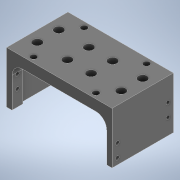
# Autodesk Inventor part: Carriage
Saved by Autodesk Inventor 2022 (Build 260153000, 153)
## iProperties
Created: 2021-06-15
Part Number: Carriage
Material: Generic
Document SubType Name: Modeling
Designer: burgessb
Density: 1 g/cm^3
Appearance: Gray
Author: burgessb
Autodesk Inventor part; units mm, degrees
ref_plane "YZ Plane" through (0, 0, 0) normal (1, 0, 0) x (0, 1, 0)
ref_plane "XZ Plane" through (0, 0, 0) normal (0, 1, 0) x (-1, 0, 0)
ref_plane "XY Plane" through (0, 0, 0) normal (0, 0, 1) x (1, 0, 0)
sketch "Sketch1" plane through (0, 0, 0) normal (0, 1, 0) x (-1, 0, 0)
  line L0 (-45, 17.5) -> (45, 17.5)
  line L1 (45, 17.5) -> (45, -17.5)
  line L2 (45, -17.5) -> (-45, -17.5)
  line L3 (-45, -17.5) -> (-45, 17.5)
  line L4 (-45, 17.5) -> (45, -17.5) construction
  line L5 (45, 17.5) -> (-45, -17.5) construction
  circle A0 centre (-39, 10) radius 2.25
  circle A1 centre (-11, 10) radius 2.25
  circle A2 centre (-11, -10) radius 2.25
  circle A3 centre (-39, -10) radius 2.25
  line L6 (0, 17.5) -> (0, -17.5) construction
  circle A4 centre (39, 10) radius 2.25
  circle A5 centre (11, 10) radius 2.25
  circle A6 centre (11, -10) radius 2.25
  circle A7 centre (39, -10) radius 2.25
  point P0 (0, 0)
  dimension "d0" = 90
  dimension "d1" = 35
  dimension "d12" = 4.5
  dimension "d13" = 4.5
  dimension "d14" = 4.5
  dimension "d15" = 4.5
  dimension "d16" = 0
  dimension "d17" = 0
  dimension "d18" = 0
  dimension "d19" = 0
  dimension "d21" = 10
  dimension "d22" = 20
  dimension "d23" = 28
  dimension "d50" = 50
  constraints: 14 end point, 8 centre point, 4 midpoint, 4 symmetric about line, 2 parallel, 1 horizontal, 1 perpendicular, 4 other
  measures "d0" distance of L1.end L2.end
  measures "d1" distance of L0.end L1.end
  measures "d12" diameter of A0
  measures "d13" diameter of A1
  measures "d14" diameter of A2
  measures "d15" diameter of A3
  measures "d16" horizontal distance of A2.centre A1.centre
  measures "d17" vertical distance of A3.centre A2.centre
  measures "d18" horizontal distance of A3.centre A0.centre
  measures "d19" vertical distance of A0.centre A1.centre
  measures "d21" vertical distance of point (0, 0) A1.centre
  measures "d22" distance of A2.centre A1.centre
  measures "d23" distance of A2.centre A3.centre
  measures "d50" distance of A6.centre A3.centre
extrude "Extrusion1" add sketch "Sketch1" along normal blind 8
sketch "Sketch2" plane through (0, 8, 0) normal (0, 1, 0) x (1, 0, 0)
  line L0 (45, 17.5) -> (-45, 17.5) projected
  line L1 (-45, 17.5) -> (-45, -17.5) projected
  line L2 (-45, -17.5) -> (45, -17.5) projected
  line L3 (45, -17.5) -> (45, 17.5) projected
  line L4 (46, -18.5) -> (-46, -18.5)
  line L5 (-46, -18.5) -> (-46, 18.5)
  line L6 (-46, 18.5) -> (46, 18.5)
  line L7 (46, 18.5) -> (46, -18.5)
  line L8 (49, -28.5) -> (49, 28.5)
  line L9 (49, -28.5) -> (44, -28.5)
  line L10 (44, -28.5) -> (44, -18.5)
  line L11 (49, 28.5) -> (44, 28.5)
  line L12 (44, 28.5) -> (44, 18.5)
  line L13 (44, -18.5) -> (44, -17.5)
  line L14 (-45, -17.5) -> (45, -17.5) projected
  line L15 (44, 18.5) -> (44, 17.5)
  line L16 (45, 17.5) -> (-45, 17.5) projected
  line L17 (0, -21.8029) -> (0, 22.7316) construction
  line L18 (-49, -28.5) -> (-49, 28.5)
  line L19 (-49, -28.5) -> (-44, -28.5)
  line L20 (-44, -28.5) -> (-44, -18.5)
  line L21 (-49, 28.5) -> (-44, 28.5)
  line L22 (-44, 28.5) -> (-44, 18.5)
  line L23 (-44, -18.5) -> (-44, -17.5)
  line L24 (-44, 18.5) -> (-44, 17.5)
  point P0 (0, 0)
  point P1 (-44, 17.5)
  dimension "d4" = 1
  dimension "d5" = 3
  dimension "d6" = 10
  dimension "d7" = 10
  dimension "d8" = 5
  dimension "d9" = 5
  dimension "d24" = 0
  constraints: 38 end point, 10 point on line, 8 symmetric about line, 2 perpendicular, 2 vertical, 1 horizontal, 3 other
  measures "d4" distance between parallel lines of L2 L4
  measures "d5" distance between parallel lines of L8 L7
  measures "d6" vertical distance of L6.end L8.end
  measures "d7" vertical distance of L4.start L8.start
  measures "d8" distance of L8.start L9.end
  measures "d9" distance of L8.end L11.end
  measures "d24" distance from line of point (0, 0) L17
extrude "Extrusion2" add sketch "Sketch2" against normal blind 8 contours L0 L15 L6 L7 L4 L13 L2 L3 | L0 L1 L2 L23 L4 L5 L6 L24 | L12 L11 L8 L9 L10 L4 L7 L6 | L6 L5 L4 L20 L19 L18 L21 L22
sketch "Sketch3" plane through (0, 0, 0) normal (0, -1, 0) x (1, 0, 0)
  line L0 (44, -17.5) -> (44, -28.5) projected
  line L1 (44, -28.5) -> (49, -28.5) projected
  line L2 (49, -28.5) -> (49, 28.5) projected
  line L3 (49, 28.5) -> (44, 28.5) projected
  line L4 (44, 28.5) -> (44, 17.5) projected
  line L5 (-44, 17.5) -> (44, 17.5) projected
  line L6 (-44, 17.5) -> (-44, 28.5) projected
  line L7 (-44, 28.5) -> (-49, 28.5) projected
  line L8 (-49, 28.5) -> (-49, -28.5) projected
  line L9 (-49, -28.5) -> (-44, -28.5) projected
  line L10 (-44, -28.5) -> (-44, -17.5) projected
  line L11 (44, -17.5) -> (-44, -17.5) projected
  circle A0 centre (-11, -10) radius 2.25 projected
  circle A1 centre (-11, 10) radius 2.25 projected
  circle A2 centre (-39, 10) radius 2.25 projected
  circle A3 centre (-39, -10) radius 2.25 projected
  circle A4 centre (39, -10) radius 2.25 projected
  circle A5 centre (11, -10) radius 2.25 projected
  circle A6 centre (11, 10) radius 2.25 projected
  circle A7 centre (39, 10) radius 2.25 projected
  line L12 (-45, -17.5) -> (45, -17.5)
  line L13 (45, -17.5) -> (45, 17.5)
  line L14 (45, 17.5) -> (-45, 17.5)
  line L15 (-45, 17.5) -> (-45, -17.5)
  line L16 (-45, -17.5) -> (45, 17.5) construction
  line L17 (45, -17.5) -> (-45, 17.5) construction
  line L18 (-46, -18.5) -> (46, -18.5)
  line L19 (46, -18.5) -> (46, 18.5)
  line L20 (46, 18.5) -> (-46, 18.5)
  line L21 (-46, 18.5) -> (-46, -18.5)
  line L22 (-44, 17.5) -> (-44, 18.5)
  line L23 (-44, -17.5) -> (-44, -18.5)
  line L24 (44, -17.5) -> (-44, -17.5) projected
  line L25 (44, -17.5) -> (44, -18.5)
  line L26 (44, 17.5) -> (44, 18.5)
  point P0 (0, 0)
  point P1 (44, 18.5)
  point P2 (44, -18.5)
  point P3 (-44, -18.5)
  point P4 (-44, 18.5)
  dimension "d26" = 35
  dimension "d27" = 1
  dimension "d52" = 90
  constraints: 28 end point, 4 parallel, 4 perpendicular, 4 point on line, 2 midpoint, 2 vertical, 1 horizontal, 3 other
  measures "d26" distance of L13.end L12.end
  measures "d27" distance between parallel lines of L15 L21
  measures "d52" distance of L13.end L14.end
extrude "Extrusion3" add sketch "Sketch3" along normal blind 30 contours L18 L19 L20 L4 L3 L2 L1 L0 | L10 L9 L8 L7 L6 L20 L21 L18
sketch "Sketch4" plane through (49, 8, 28.5) normal (1, 0, 0) x (0, 0, -1)
  circle A0 centre (5, -32.5) radius 1.65
  circle A1 centre (5, -20.5) radius 1.65
  line L0 (0, 0) -> (57, 0) projected
  line L1 (0, 0) -> (0, -38) projected
  line L2 (57, 0) -> (57, -38) projected
  circle A2 centre (52, -23.5) radius 1.65
  circle A3 centre (52, -11.5) radius 1.65
  line L3 (57, -38) -> (0, -38) projected
  line L4 (16.25, -8) -> (20.75, -8) projected
  line L5 (16.25, -8) -> (20.75, -8) projected
  line L6 (36.25, -8) -> (40.75, -8) projected
  line L7 (36.25, -8) -> (40.75, -8) projected
  line L8 (36.25, -8) -> (40.75, -8) projected
  line L9 (16.25, -8) -> (20.75, -8) projected
  line L10 (16.25, -8) -> (20.75, -8) projected
  line L11 (36.25, -8) -> (40.75, -8) projected
  line L12 (47, -8) -> (10, -8) projected
  line L13 (10, -8) -> (11, -8) projected
  line L14 (11, -8) -> (10, -8) projected
  line L15 (10, -8) -> (47, -8) projected
  line L16 (47, -8) -> (46, -8) projected
  line L17 (46, -8) -> (47, -8) projected
  line L18 (19.0432, -26.5) -> (-6.642, -26.5)
  point P0 (28.5, -8)
  dimension "d30" = 3.3
  dimension "d31" = 3.3
  dimension "d33" = 12
  dimension "d34" = 0
  dimension "d36" = 5
  dimension "d39" = 3.3
  dimension "d40" = 3.3
  dimension "d41" = 12
  dimension "d42" = 0
  dimension "d43" = 5
  dimension "d53" = 9
  dimension "d54" = 18.5
  dimension "d55" = 6
  dimension "d56" = 6
  constraints: 4 centre point, 2 end point, 1 horizontal
  measures "d30" diameter of A0
  measures "d31" diameter of A1
  measures "d33" distance of A0.centre A1.centre
  measures "d34" horizontal distance of A0.centre A1.centre
  measures "d36" distance from line of L1 A0.centre
  measures "d39" diameter of A2
  measures "d40" diameter of A3
  measures "d41" distance of A2.centre A3.centre
  measures "d42" horizontal distance of A2.centre A3.centre
  measures "d43" distance from line of L2 A2.centre
  measures "d53" vertical distance of A3.centre A1.centre
  measures "d54" distance between parallel lines of L18 L12
  measures "d55" distance from line of L18 A1.centre
  measures "d56" distance from line of L18 A0.centre
extrude "Extrusion4" cut sketch "Sketch4" against normal up to surface (5 mm away) contours A0 | A1 | A2 | A3
sketch "Sketch5" plane through (-49, 8, -28.5) normal (-1, 0, 0) x (0, 0, 1)
  line L0 (0, 0) -> (11, 0) projected
  line L1 (0, 0) -> (0, -38) projected
  line L2 (11, 0) -> (11, -8) projected
  line L3 (46, 0) -> (57, 0) projected
  line L4 (46, -8) -> (46, 0) projected
  line L5 (57, 0) -> (57, -38) projected
  line L6 (57, 0) -> (0, 0) projected
  line L7 (28.5, 0) -> (28.5, -38) construction
  line L8 (57, -38) -> (0, -38) projected
  line L9 (47, -8) -> (46, -8) projected
  line L10 (11, -8) -> (10, -8) projected
  line L11 (57, -38) -> (47, -38) projected
  line L12 (10, -38) -> (0, -38) projected
  line L13 (47, -8) -> (47, -38) projected
  line L14 (10, -8) -> (10, -38) projected
  circle A0 centre (5, -23.5) radius 1.65 projected
  circle A1 centre (5, -23.5) radius 1.65 projected
  circle A2 centre (5, -11.5) radius 1.65 projected
  circle A3 centre (5, -11.5) radius 1.65 projected
  circle A4 centre (52, -32.5) radius 1.65 projected
  circle A5 centre (52, -32.5) radius 1.65 projected
  circle A6 centre (52, -20.5) radius 1.65 projected
  circle A7 centre (52, -20.5) radius 1.65 projected
  circle A8 centre (52, -23.5) radius 1.65
  circle A9 centre (52, -23.5) radius 1.65
  circle A10 centre (52, -11.5) radius 1.65
  circle A11 centre (52, -11.5) radius 1.65
  circle A12 centre (5, -32.5) radius 1.65
  circle A13 centre (5, -32.5) radius 1.65
  circle A14 centre (5, -20.5) radius 1.65
  circle A15 centre (5, -20.5) radius 1.65
  point P0 (28.5, -8)
  point P1 (10, -35)
  point P2 (42, -35)
  point P3 (51.3126, -22)
  point P4 (52.6874, -22)
  point P5 (5.6874, -22)
  point P6 (4.3126, -22)
  constraints: 8 centre point, 8 symmetric about line, 2 end point, 1 midpoint, 10 other
extrude "Extrusion5" cut sketch "Sketch5" against normal up to surface (5 mm away) contours A14 A0 | A0 A14 | A8 A6 | A6 A8 | A10 | A12 picked at (4.8827, -21.9626) picked at (5.0265, -19.8581) picked at (51.8827, -22.0374) picked at (52.0265, -24.1419)
sketch "Sketch6" plane through (0, 8, 0) normal (0, 1, 0) x (1, 0, 0)
  line L0 (44, 17.5) -> (-44, 17.5) projected
  line L1 (-44, 17.5) -> (-44, 28.5) projected
  line L2 (-44, 28.5) -> (-49, 28.5) projected
  line L3 (-49, 28.5) -> (-49, -28.5) projected
  line L4 (-49, -28.5) -> (-44, -28.5) projected
  line L5 (-44, -28.5) -> (-44, -17.5) projected
  line L6 (-44, -17.5) -> (44, -17.5) projected
  line L7 (44, -17.5) -> (44, -28.5) projected
  line L8 (44, -28.5) -> (49, -28.5) projected
  line L9 (49, -28.5) -> (49, 28.5) projected
  line L10 (49, 28.5) -> (44, 28.5) projected
  line L11 (44, 28.5) -> (44, 17.5) projected
  circle A0 centre (-11, 10) radius 2.25 projected
  circle A1 centre (-11, -10) radius 2.25 projected
  circle A2 centre (-39, -10) radius 2.25 projected
  circle A3 centre (-39, 10) radius 2.25 projected
  circle A4 centre (39, 10) radius 2.25 projected
  circle A5 centre (11, 10) radius 2.25 projected
  circle A6 centre (11, -10) radius 2.25 projected
  circle A7 centre (39, -10) radius 2.25 projected
  line L12 (-44, -17.5) -> (-44, -28.5) projected
  line L13 (44, -28.5) -> (49, -28.5) projected
  line L14 (-44, -28.5) -> (44, -28.5)
  line L15 (44, 28.5) -> (44, 17.5) projected
  line L16 (44, 28.5) -> (-44, 28.5)
  point P0 (0, 0)
  point P1 (-44, -18.5)
  constraints: 4 end point, 1 collinear, 1 perpendicular
extrude "Extrusion6" add sketch "Sketch6" against normal blind 8 contours L0 L1 L16 L11 | L14 L5 L6 L7
sketch "Sketch10" plane through (0, 8, 0) normal (0, 1, 0) x (1, 0, 0)
  line L0 (49, 28.5) -> (-49, 28.5) projected
  line L1 (-49, 28.5) -> (-49, -28.5) projected
  line L2 (-49, -28.5) -> (49, -28.5) projected
  line L3 (49, -28.5) -> (49, 28.5) projected
  circle A0 centre (-11, 10) radius 2.25 projected
  circle A1 centre (-11, -10) radius 2.25 projected
  circle A2 centre (-39, -10) radius 2.25 projected
  circle A3 centre (-39, 10) radius 2.25 projected
  circle A4 centre (39, 10) radius 2.25 projected
  circle A5 centre (11, 10) radius 2.25 projected
  circle A6 centre (11, -10) radius 2.25 projected
  circle A7 centre (39, -10) radius 2.25 projected
  circle A8 centre (39, -10) radius 4
  circle A9 centre (11, -10) radius 4
  circle A10 centre (-11, -10) radius 2.25 projected
  circle A11 centre (-11, -10) radius 4
  circle A12 centre (-39, -10) radius 2.25 projected
  circle A13 centre (-39, -10) radius 4
  circle A14 centre (-39, 10) radius 2.25 projected
  circle A15 centre (-39, 10) radius 4
  circle A16 centre (-11, 10) radius 4
  circle A17 centre (11, 10) radius 2.25 projected
  circle A18 centre (11, 10) radius 4
  circle A19 centre (39, 10) radius 4
  point P0 (0, 0)
  dimension "d81" = 8
  constraints: 8 centre point, 8 coincident, 7 equal radius
  measures "d81" diameter of A8
extrude "Extrusion10" add sketch "Sketch10" along normal blind 10 contours L3 L2 L1 L0
sketch "Sketch11" plane through (0, 0, 0) normal (0, -1, 0) x (1, 0, 0)
  circle A0 centre (39, 10) radius 2.25 projected
  circle A1 centre (11, 10) radius 2.25 projected
  circle A2 centre (11, -10) radius 2.25 projected
  circle A3 centre (39, -10) radius 2.25 projected
  circle A4 centre (-39, -10) radius 2.25 projected
  circle A5 centre (-39, 10) radius 2.25 projected
  circle A6 centre (-11, 10) radius 2.25 projected
  circle A7 centre (-11, -10) radius 2.25 projected
  line L0 (44, -18.5) -> (46, -18.5) projected
  line L1 (46, -18.5) -> (46, 18.5) projected
  line L2 (46, 18.5) -> (44, 18.5) projected
  line L3 (44, 28.5) -> (44, 18.5) projected
  line L4 (44, 28.5) -> (-44, 28.5) projected
  line L5 (-44, 18.5) -> (-44, 28.5) projected
  line L6 (-44, 18.5) -> (-46, 18.5) projected
  line L7 (-46, 18.5) -> (-46, -18.5) projected
  line L8 (-46, -18.5) -> (-44, -18.5) projected
  line L9 (-44, -28.5) -> (-44, -18.5) projected
  line L10 (-44, -28.5) -> (44, -28.5) projected
  line L11 (44, -18.5) -> (44, -28.5) projected
  line L12 (44, -18.5) -> (-44, -18.5)
  line L13 (46, 18.5) -> (46, -18.5) projected
  line L14 (-46, 18.5) -> (-44, 18.5) projected
  line L15 (-44, 18.5) -> (44, 18.5)
  point P0 (0, 0)
  constraints: 4 end point, 1 collinear, 1 perpendicular
extrude "Extrusion11" cut sketch "Sketch11" against normal blind 8 contours L11 L10 L9 L12 | L15 L5 L4 L3
fillet "Fillet8" radius 10 4 edges at (-44, 8, 23.5) (44, 8, 23.5) (44, 8, -23.5) (-44, 8, -23.5)
sketch "Sketch12" plane through (0, 8, 0) normal (0, -1, 0) x (1, 0, 0)
  line L0 (34, 28.5) -> (34, 18.5) projected
  line L1 (-34, 28.5) -> (34, 28.5) projected
  line L2 (-34, 18.5) -> (-34, 28.5) projected
  line L3 (34, 18.5) -> (-34, 18.5) projected
  line L4 (-34, -28.5) -> (-34, -18.5) projected
  line L5 (34, -28.5) -> (-34, -28.5) projected
  line L6 (34, -18.5) -> (34, -28.5) projected
  line L7 (-34, -18.5) -> (34, -18.5) projected
  circle A0 centre (-29, 23.5) radius 2.75
  circle A1 centre (29, 23.5) radius 2.75
  circle A2 centre (-29, -23.5) radius 2.75
  circle A3 centre (29, -23.5) radius 2.75
  point P0 (0, 0)
  dimension "d89" = 5.5
  dimension "d90" = 5
  dimension "d91" = 5
  dimension "d92" = 68
  dimension "d93" = 57
  dimension "d96" = 58
  dimension "d99" = 47
  constraints: 4 centre point, 1 horizontal, 1 vertical, 6 other
  measures "d89" diameter of A0
  measures "d90" distance from line of L1 A0.centre
  measures "d91" distance from line of L2 A0.centre
  measures "d92" distance between parallel lines of L0 L2
  measures "d93" distance between parallel lines of L5 L1
  measures "d96" distance of A0.centre A1.centre
  measures "d99" distance of A0.centre A2.centre
extrude "Extrusion12" cut sketch "Sketch12" against normal through all contours A0 | A1 | A2 | A3
fillet "Fillet9" radius 2 6 edges at (40.3246, 5.746, -18.5) (-40.3246, 5.746, -18.5) (0, 8, -18.5) (-40.3246, 5.746, 18.5) (40.3246, 5.746, 18.5) (0, 8, 18.5)
equation "\"d21\" = 0.5 * d22"
equation "\"d30\" = d31"
equation "\"d39\" = d31"
equation "\"d40\" = d31"
equation "\"d41\" = d33"
equation "\"d43\" = d36"
equation "\"d55\" = d56"
body "Solid1"
